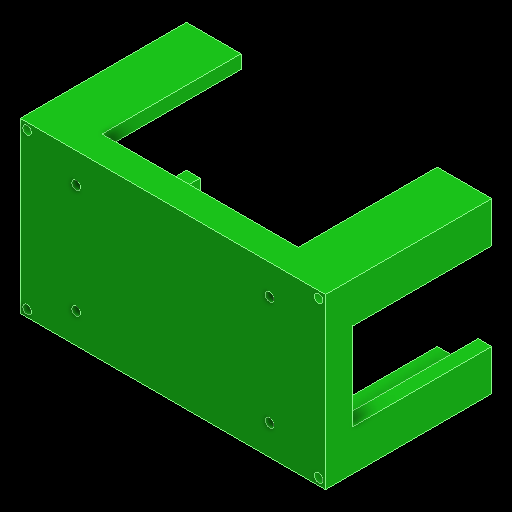
# Autodesk Inventor part: magnet_holder
Saved by Autodesk Inventor 2026.1 (Build 301233000, 233)
## iProperties
Created: 2025-09-30
Part Number: magnet_holder
Material: PC/ABS Plastic
Document SubType Name: Modeling
Designer: drago
Density: 1.1 g/cm^3
Appearance: Dark Green
Author: drago
Autodesk Inventor part; units mm, degrees
ref_plane "YZ Plane" through (0, 0, 0) normal (1, 0, 0) x (0, 1, 0)
ref_plane "XZ Plane" through (0, 0, 0) normal (0, 1, 0) x (-1, 0, 0)
ref_plane "XY Plane" through (0, 0, 0) normal (0, 0, 1) x (1, 0, 0)
sketch "Sketch1" plane through (0, 0, 0) normal (0, 0, 1) x (1, 0, 0)
  line L0 (56, -31) -> (-56, -31)
  line L1 (-56, -31) -> (-56, 31)
  line L2 (-56, 31) -> (56, 31)
  line L3 (56, 31) -> (56, -31)
  line L4 (51, -26) -> (-51, -26)
  line L5 (-51, -26) -> (-51, 26)
  line L6 (-51, 26) -> (51, 26)
  line L7 (51, 26) -> (51, -26)
  line L8 (56, 0) -> (-56, 0) construction
  line L9 (0, -31) -> (0, 31) construction
  line L10 (-36, 31) -> (-36, 26)
  line L11 (-56, 16) -> (-51, 16)
  line L12 (36, -26) -> (36, -31)
  line L13 (51, -16) -> (56, -16)
  line L14 (-36, -26) -> (-36, -31)
  line L15 (-56, -16) -> (-51, -16)
  line L16 (36, 31) -> (36, 26)
  line L17 (51, 16) -> (56, 16)
  line L18 (-53.5, 28.5) -> (53.5, 28.5) construction
  line L19 (53.5, 28.5) -> (53.5, -28.5) construction
  line L20 (53.5, -28.5) -> (-53.5, -28.5) construction
  line L21 (-53.5, -28.5) -> (-53.5, 28.5) construction
  line L22 (-53.5, 28.5) -> (53.5, -28.5) construction
  line L23 (53.5, 28.5) -> (-53.5, -28.5) construction
  point P0 (0, 0)
  point P1 (-35.5, 20)
  point P2 (35.5, 20)
  point P3 (35.5, -20)
  point P4 (-35.5, -20)
  dimension "d0" = 112
  dimension "d1" = 62
  dimension "d2" = 102
  dimension "d3" = 52
  dimension "d4" = 15
  dimension "d5" = 20
  dimension "d6" = 40
  dimension "d7" = 71
  constraints: 48 end point, 16 point on line, 12 perpendicular, 6 midpoint, 6 parallel, 4 coincident, 4 collinear, 3 horizontal, 3 symmetric about line, 7 other
  measures "d0" distance of L1.end L2.end
  measures "d1" distance between parallel lines of L0 L2
  measures "d2" distance of L5.end L6.end
  measures "d3" distance of L4.end L5.end
  measures "d4" distance between parallel lines of L0 L13
  measures "d5" distance between parallel lines of L3 L12
  measures "d6" distance of point (35.5, 20) point (35.5, -20)
  measures "d7" distance of point (35.5, -20) point (-35.5, -20)
extrude "Extrusion4" add sketch "Sketch1" against normal blind 51 contours L0 L12 L4 L7 L13 L3 | L0 L1 L15 L5 L4 L14 | L17 L7 L6 L16 L2 L3 | L1 L2 L10 L6 L5 L11
extrude "Extrusion5" add sketch "Sketch1" along normal blind 10
hole "Hole4" at (53.5, 28.5, 0) at (-53.5, -28.5, 0) at (53.5, -28.5, 0) at (-53.5, 28.5, 0) direction (0, 0, 1) diameter 3.2 end through all both
hole "Hole5" at (-35.5, 20, 0) at (35.5, 20, 0) at (35.5, -20, 0) at (-35.5, -20, 0) direction (0, 0, 1) diameter 3.2 end through all counterbore diameter 5 counterbore depth 5
equation "\"d0\" = delta + magnet_length + epsilon"
equation "\"d1\" = delta + magnet_width + epsilon"
equation "\"d2\" = magnet_length + epsilon"
equation "\"d3\" = magnet_width + epsilon"
equation "\"d35\" = 0.5 * epsilon + 0.5 * magnet_length"
equation "\"magnet_width\" = 50"
equation "\"magnet_length\" = 100"
equation "\"delta\" = 10"
equation "\"epsilon\" = 2"
body "Solid2"
